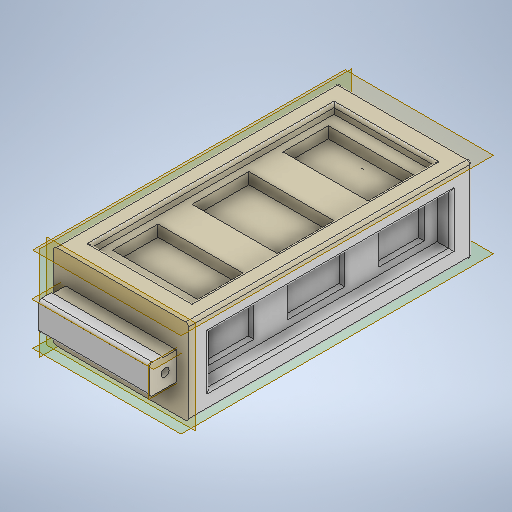
# Autodesk Inventor part: Part7
Saved by Autodesk Inventor 2025.2 (Build 292293000, 293)
## iProperties
Created: 2024-12-22
Part Number: Part7
Material: 一般
Document SubType Name: Modeling
Designer: mahhy
Density: 1 g/cm^3
Appearance: 既定
Author: mahhy
## iProperties of the stored document Part7_3D プリント.ipt
Created: 2024-12-23
Part Number: Part7_3D プリント
Material: 一般
Document SubType Name: Modeling
Designer: mahhy
Density: 1 g/cm^3
Appearance: 既定
Author: mahhy
Autodesk Inventor part; units mm, degrees
ref_plane "YZ Plane" through (0, 0, 0) normal (1, 0, 0) x (0, 1, 0)
ref_plane "XZ Plane" through (0, 0, 0) normal (0, 1, 0) x (-1, 0, 0)
ref_plane "XY Plane" through (0, 0, 0) normal (0, 0, 1) x (1, 0, 0)
sketch "スケッチ1" plane through (0, 0, 0) normal (0, 1, 0) x (-1, 0, 0)
  line L0 (0, 0) -> (47.5, 0)
  line L1 (47.5, 0) -> (47.5, -100)
  line L2 (47.5, -100) -> (0, -100)
  line L3 (0, -100) -> (0, 0)
  dimension "d0" = 47.5
  dimension "d1" = 100
  constraints: 8 end point, 2 parallel, 1 horizontal, 1 perpendicular
  measures "d0" distance of L1.end L2.end
  measures "d1" distance of L0.end L1.end
extrude "押し出し1" add sketch "スケッチ1" along normal blind 30
ref_plane "作業平面1" through (-47.5, 0, 0) normal (0, 0, 1) x (1, 0, 0)
sketch "スケッチ2" plane through (-47.5, 0, 0) normal (0, 0, 1) x (1, 0, 0)
  line L0 (4.25, 19.88) -> (43.25, 19.88)
  line L1 (43.25, 19.88) -> (43.25, 10.12)
  line L2 (43.25, 10.12) -> (4.25, 10.12)
  line L3 (4.25, 10.12) -> (4.25, 19.88)
  line L4 (47.5, 0) -> (0, 0) projected
  line L5 (0, 0) -> (47.5, 0) projected
  line L6 (0, 0) -> (0, 30) projected
  line L7 (0, 0) -> (0, 30) projected
  point P0 (23.75, 10.12)
  point P1 (23.75, 0)
  point P2 (23.75, 0)
  point P3 (4.25, 15)
  point P4 (0, 15)
  point P5 (0, 15)
  dimension "d5" = 39
  dimension "d6" = 9.76
  dimension "d7" = 0
  dimension "d8" = 0
  constraints: 8 end point, 6 midpoint, 2 parallel, 1 horizontal, 1 perpendicular
  measures "d5" distance of L1.end L2.end
  measures "d6" distance of L0.end L1.end
  measures "d7" horizontal distance of point (23.75, 0) point (23.75, 10.12)
  measures "d8" vertical distance of point (0, 15) point (4.25, 15)
extrude "押し出し2" add sketch "スケッチ2" along normal blind 9.5
ref_plane "作業平面2" through (-4.25, 10.12, 0) normal (1, 0, 0) x (0, 0, -1)
sketch "スケッチ3" plane through (-4.25, 10.12, 0) normal (1, 0, 0) x (0, 0, -1)
  line L0 (-9.5, 0) -> (-9.5, 9.76) projected
  line L1 (0, -10.12) -> (0, 19.88) projected
  point P0 (-9.5, 4.88)
  point P1 (-4, 4.88)
  point P2 (0, 4.88)
  dimension "d12" = 4
  constraints: 2 midpoint
  measures "d12" distance of point (0, 4.88) point (-4, 4.88)
hole "穴1" at (-4.25, 15, 4) direction (-1, 0, 0) diameter 2.85 end through all
ref_plane "作業平面3" through (-43.25, 19.88, 0) normal (0, 1, 0) x (1, 0, 0)
sketch "スケッチ4" plane through (-43.25, 19.88, 0) normal (0, 1, 0) x (1, 0, 0)
  line L0 (0, 0) -> (0, -9.5) projected
  line L1 (0, -9.5) -> (39, -9.5)
  line L2 (39, -9.5) -> (39, -5)
  line L3 (39, -5) -> (0, -5)
  line L4 (0, -5) -> (0, -9.5)
  point P0 (43.25, 0)
  dimension "d21" = 4.5
  constraints: 8 end point, 2 parallel, 1 horizontal, 1 perpendicular
  measures "d21" distance of L2.end L1.end
extrude "押し出し3" add sketch "スケッチ4" along normal blind 0.5
ref_plane "作業平面4" through (0, 30, 0) normal (0, 1, 0) x (1, 0, 0)
sketch "スケッチ6" plane through (0, 30, 0) normal (0, 1, 0) x (1, 0, 0)
  line L0 (-38.75, 28) -> (-8.75, 28)
  line L1 (-8.75, 28) -> (-8.75, 12)
  line L2 (-8.75, 12) -> (-38.75, 12)
  line L3 (-38.75, 12) -> (-38.75, 28)
  line L4 (-4.25, 0) -> (-43.25, 0) projected
  line L5 (9.5, 0) -> (-57, 0) projected
  line L6 (-38.75, 60) -> (-8.75, 60)
  line L7 (-8.75, 60) -> (-8.75, 40)
  line L8 (-8.75, 40) -> (-38.75, 40)
  line L9 (-38.75, 40) -> (-38.75, 60)
  line L10 (-38.75, 88) -> (-8.75, 88)
  line L11 (-8.75, 88) -> (-8.75, 72)
  line L12 (-8.75, 72) -> (-38.75, 72)
  line L13 (-38.75, 72) -> (-38.75, 88)
  line L14 (0, 100) -> (-47.5, 100) projected
  point P0 (0, 0)
  point P1 (-23.75, 12)
  point P2 (-23.75, 0)
  point P3 (-23.75, 40)
  point P4 (-23.75, 72)
  point P5 (-23.75, 60)
  point P6 (-23.75, 28)
  dimension "d37" = 30
  dimension "d38" = 16
  dimension "d39" = 0
  dimension "d40" = 12
  dimension "d41" = 30
  dimension "d42" = 20
  dimension "d43" = 30
  dimension "d44" = 16
  dimension "d45" = 12
  dimension "d46" = 12
  dimension "d47" = 12
  dimension "d48" = 0
  dimension "d49" = 0
  constraints: 24 end point, 6 midpoint, 6 parallel, 3 horizontal, 3 perpendicular
  measures "d37" distance of L1.end L2.end
  measures "d38" distance of L0.end L1.end
  measures "d39" horizontal distance of point (-23.75, 0) point (-23.75, 12)
  measures "d40" distance between parallel lines of L5 L2
  measures "d41" distance of L7.end L8.end
  measures "d42" distance of L6.end L7.end
  measures "d43" distance of L11.end L12.end
  measures "d44" distance of L10.end L11.end
  measures "d45" distance between parallel lines of L0 L8
  measures "d46" distance between parallel lines of L12 L6
  measures "d47" distance between parallel lines of L14 L10
  measures "d48" horizontal distance of point (-23.75, 60) point (-23.75, 72)
  measures "d49" horizontal distance of point (-23.75, 28) point (-23.75, 40)
extrude "押し出し5" cut sketch "スケッチ6" against normal blind 7
ref_plane "作業平面5" through (0, 0, 0) normal (0, -1, 0) x (1, 0, 0)
sketch "スケッチ7" plane through (0, 0, 0) normal (0, -1, 0) x (1, 0, 0)
  line L0 (-38.75, -72) -> (-8.75, -72)
  line L1 (-8.75, -72) -> (-8.75, -88)
  line L2 (-8.75, -88) -> (-38.75, -88)
  line L3 (-38.75, -88) -> (-38.75, -72)
  line L4 (-38.75, -40) -> (-8.75, -40)
  line L5 (-8.75, -40) -> (-8.75, -60)
  line L6 (-8.75, -60) -> (-38.75, -60)
  line L7 (-38.75, -60) -> (-38.75, -40)
  line L8 (-38.75, -12) -> (-8.75, -12)
  line L9 (-8.75, -12) -> (-8.75, -28)
  line L10 (-8.75, -28) -> (-38.75, -28)
  line L11 (-38.75, -28) -> (-38.75, -12)
  line L12 (-47.5, 0) -> (0, 0) projected
  point P0 (-23.75, -88)
  point P1 (-23.75, -60)
  point P2 (-23.75, -28)
  point P3 (-23.75, -40)
  point P4 (-23.75, -72)
  point P5 (-23.75, 0)
  point P6 (-23.75, -12)
  dimension "d53" = 30
  dimension "d54" = 16
  dimension "d55" = 30
  dimension "d56" = 20
  dimension "d57" = 30
  dimension "d58" = 16
  dimension "d59" = 12
  dimension "d60" = 12
  dimension "d61" = 0
  dimension "d62" = 0
  dimension "d63" = 0
  dimension "d64" = 12
  constraints: 24 end point, 7 midpoint, 6 parallel, 3 horizontal, 3 perpendicular
  measures "d53" distance of L1.end L3.start
  measures "d54" distance of L0.end L1.end
  measures "d55" distance of L6.start L6.end
  measures "d56" distance of L5.start L6.start
  measures "d57" distance of L10.start L10.end
  measures "d58" distance of L9.start L10.start
  measures "d59" distance between parallel lines of L0 L6
  measures "d60" distance between parallel lines of L10 L4
  measures "d61" horizontal distance of point (-23.75, -40) point (-23.75, -28)
  measures "d62" horizontal distance of point (-23.75, -72) point (-23.75, -60)
  measures "d63" horizontal distance of point (-23.75, 0) point (-23.75, -12)
  measures "d64" distance between parallel lines of L12 L8
extrude "押し出し6" cut sketch "スケッチ7" against normal blind 7
sketch "スケッチ8" plane through (0, 30, 0) normal (0, 1, 0) x (1, 0, 0)
  line L0 (-41.25, 92.5) -> (-6.25, 92.5)
  line L1 (-6.25, 92.5) -> (-6.25, 7.5)
  line L2 (-6.25, 7.5) -> (-41.25, 7.5)
  line L3 (-41.25, 7.5) -> (-41.25, 92.5)
  line L4 (0, 100) -> (-47.5, 100) projected
  line L5 (-47.5, 100) -> (-47.5, 0) projected
  line L6 (0, 0) -> (0, 100) projected
  point P0 (-23.75, 92.5)
  point P1 (-23.75, 100)
  point P2 (-41.25, 50)
  point P3 (-47.5, 50)
  dimension "d67" = 35
  dimension "d68" = 85
  dimension "d69" = 0
  dimension "d70" = 0
  dimension "d120" = 7.5
  dimension "d121" = 6.25
  constraints: 8 end point, 4 midpoint, 2 parallel, 1 horizontal, 1 perpendicular
  measures "d67" distance of L1.end L2.end
  measures "d68" distance of L0.end L1.end
  measures "d69" horizontal distance of point (-23.75, 100) point (-23.75, 92.5)
  measures "d70" vertical distance of point (-47.5, 50) point (-41.25, 50)
  measures "d120" distance between parallel lines of L4 L0
  measures "d121" distance between parallel lines of L6 L1
extrude "押し出し7" cut sketch "スケッチ8" against normal blind 3
sketch "スケッチ9" plane through (0, 0, 0) normal (0, -1, 0) x (1, 0, 0)
  line L0 (-6.25, -7.5) -> (-41.25, -7.5) projected
  line L1 (-6.25, -92.5) -> (-6.25, -7.5) projected
  line L2 (-41.25, -7.5) -> (-6.25, -7.5)
  line L3 (-6.25, -7.5) -> (-6.25, -92.5)
  line L4 (-6.25, -92.5) -> (-41.25, -92.5)
  line L5 (-41.25, -92.5) -> (-41.25, -7.5)
  point P0 (0, 0)
  constraints: 8 end point, 2 parallel, 1 horizontal, 1 perpendicular
extrude "押し出し8" cut sketch "スケッチ9" against normal blind 5
sketch "スケッチ10" plane through (0, 0, 0) normal (1, 0, 0) x (0, 0, -1)
  line L0 (0, 0) -> (100, 0) projected
  line L1 (0, 30) -> (100, 30) projected
  line L2 (100, 0) -> (100, 30) projected
  line L3 (0, 0) -> (0, 30) projected
  line L4 (88, 21.25) -> (72, 21.25)
  line L5 (72, 21.25) -> (72, 8.75)
  line L6 (72, 8.75) -> (88, 8.75)
  line L7 (88, 8.75) -> (88, 21.25)
  line L8 (60, 21.25) -> (40, 21.25)
  line L9 (40, 21.25) -> (40, 8.75)
  line L10 (40, 8.75) -> (60, 8.75)
  line L11 (60, 8.75) -> (60, 21.25)
  line L12 (28, 21.25) -> (12, 21.25)
  line L13 (12, 21.25) -> (12, 8.75)
  line L14 (12, 8.75) -> (28, 8.75)
  line L15 (28, 8.75) -> (28, 21.25)
  point P0 (100, 15)
  point P1 (12, 15)
  point P2 (80, 21.25)
  point P3 (50, 30)
  dimension "d82" = 16
  dimension "d83" = 20
  dimension "d84" = 16
  dimension "d85" = 12
  dimension "d86" = 12
  dimension "d87" = 12
  dimension "d88" = 12
  dimension "d90" = 8.75
  dimension "d91" = 8.75
  dimension "d92" = 8.75
  dimension "d93" = 8.75
  dimension "d94" = 8.75
  dimension "d95" = 8.75
  constraints: 24 end point, 6 parallel, 4 midpoint, 3 horizontal, 3 perpendicular
  measures "d82" distance of L6.end L5.end
  measures "d83" distance of L9.end L10.end
  measures "d84" distance of L13.end L14.end
  measures "d85" distance between parallel lines of L2 L7
  measures "d86" distance between parallel lines of L15 L9
  measures "d87" distance between parallel lines of L5 L11
  measures "d88" distance from line of L3 point (12, 15)
  measures "d90" distance from line of L1 point (80, 21.25)
  measures "d91" distance between parallel lines of L0 L6
  measures "d92" distance from line of point (50, 30) L8
  measures "d93" distance between parallel lines of L0 L10
  measures "d94" distance between parallel lines of L1 L12
  measures "d95" distance between parallel lines of L0 L14
extrude "押し出し9" cut sketch "スケッチ10" against normal blind 7 contours L7 L6 L5 L4 | L11 L10 L9 L8 | L15 L14 L13 L12
ref_plane "作業平面6" through (-47.5, 0, -100) normal (-1, 0, 0) x (0, 0, 1)
sketch "スケッチ12" plane through (-47.5, 0, -100) normal (-1, 0, 0) x (0, 0, 1)
  line L0 (88, 21.43) -> (72, 21.43)
  line L1 (72, 21.43) -> (72, 8.57)
  line L2 (72, 8.57) -> (88, 8.57)
  line L3 (88, 8.57) -> (88, 21.43)
  line L4 (60, 21.43) -> (40, 21.43)
  line L5 (40, 21.43) -> (40, 8.57)
  line L6 (40, 8.57) -> (60, 8.57)
  line L7 (60, 8.57) -> (60, 21.43)
  line L8 (28, 21.43) -> (12, 21.43)
  line L9 (12, 21.43) -> (12, 8.57)
  line L10 (12, 8.57) -> (28, 8.57)
  line L11 (28, 8.57) -> (28, 21.43)
  line L12 (0, 0) -> (0, 30) projected
  line L13 (-21.9, 30) -> (131.4, 30) projected
  line L14 (131.4, 0) -> (-21.9, 0) projected
  point P0 (100, 0)
  point P1 (12, 15)
  point P2 (80, 21.43)
  point P3 (0, 15)
  point P4 (0, 15)
  point P5 (40, 15)
  point P6 (72, 15)
  dimension "d101" = 16
  dimension "d102" = 20
  dimension "d103" = 16
  dimension "d104" = 12
  dimension "d105" = 12
  dimension "d106" = 0
  dimension "d107" = 0
  dimension "d108" = 0
  dimension "d109" = 12
  dimension "d111" = 8.57
  dimension "d112" = 8.57
  dimension "d113" = 8.57
  dimension "d114" = 8.57
  constraints: 24 end point, 6 midpoint, 6 parallel, 3 horizontal, 3 perpendicular
  measures "d101" distance of L2.end L1.end
  measures "d102" distance of L6.start L6.end
  measures "d103" distance of L9.end L11.start
  measures "d104" distance between parallel lines of L11 L5
  measures "d105" distance between parallel lines of L1 L7
  measures "d106" vertical distance of point (0, 15) point (12, 15)
  measures "d107" vertical distance of point (0, 15) point (40, 15)
  measures "d108" vertical distance of point (40, 15) point (72, 15)
  measures "d109" distance between parallel lines of L12 L9
  measures "d111" distance between parallel lines of L13 L8
  measures "d112" distance between parallel lines of L14 L10
  measures "d113" distance between parallel lines of L13 L4
  measures "d114" distance between parallel lines of L13 L0
extrude "押し出し11" cut sketch "スケッチ12" against normal blind 7
sketch "スケッチ14" plane through (-47.5, 0, -100) normal (-1, 0, 0) x (0, 0, 1)
  line L0 (7.5, 6.25) -> (92.5, 6.25)
  line L1 (92.5, 6.25) -> (92.5, 23.75)
  line L2 (92.5, 23.75) -> (7.5, 23.75)
  line L3 (7.5, 23.75) -> (7.5, 6.25)
  line L4 (0, 0) -> (0, 30) projected
  line L5 (100, 36) -> (100, -6) projected
  line L6 (-21.9, 30) -> (131.4, 30) projected
  line L7 (131.4, 0) -> (-21.9, 0) projected
  point P0 (100, 0)
  dimension "d127" = 7.5
  dimension "d128" = 7.5
  dimension "d129" = 6.25
  dimension "d130" = 6.25
  constraints: 8 end point, 2 parallel, 1 horizontal, 1 perpendicular
  measures "d127" distance between parallel lines of L4 L3
  measures "d128" distance between parallel lines of L5 L1
  measures "d129" distance between parallel lines of L6 L2
  measures "d130" distance between parallel lines of L7 L0
extrude "押し出し13" cut sketch "スケッチ14" against normal blind 5 contours L3 L2 L1 L0
sketch "スケッチ15" plane through (0, 0, 0) normal (1, 0, 0) x (0, 0, -1)
  line L0 (7.5, 23.75) -> (92.5, 23.75)
  line L1 (92.5, 23.75) -> (92.5, 6.25)
  line L2 (92.5, 6.25) -> (7.5, 6.25)
  line L3 (7.5, 6.25) -> (7.5, 23.75)
  line L4 (0, 0) -> (0, 30) projected
  line L5 (100, 0) -> (100, 30) projected
  line L6 (0, 30) -> (100, 30) projected
  line L7 (0, 0) -> (100, 0) projected
  dimension "d133" = 7.5
  dimension "d134" = 7.5
  dimension "d135" = 6.25
  dimension "d136" = 6.25
  constraints: 8 end point, 2 parallel, 1 horizontal, 1 perpendicular
  measures "d133" distance between parallel lines of L4 L3
  measures "d134" distance between parallel lines of L5 L1
  measures "d135" distance between parallel lines of L6 L0
  measures "d136" distance between parallel lines of L7 L2
extrude "押し出し14" cut sketch "スケッチ15" against normal blind 5 contours L0 L1 L2 L3
sketch "スケッチ16" plane through (0, 0, -100) normal (0, 0, -1) x (-1, 0, 0)
  line L0 (41.25, 0) -> (6.25, 0) projected
  line L1 (47.5, 0) -> (47.5, 30) projected
  circle A0 centre (23.75, 15) radius 1.75
  line L2 (0, 0) -> (47.5, 0) projected
  point P0 (23.75, 0)
  point P1 (47.5, 15)
  point P2 (23.75, 0)
  dimension "d139" = 3.5
  dimension "d153" = 0
  dimension "d154" = 0
  constraints: 3 midpoint, 1 centre point, 1 coincident
  measures "d139" diameter of A0
  measures "d153" vertical distance of A0.centre point (47.5, 15)
  measures "d154" horizontal distance of point (23.75, 0) A0.centre
extrude "押し出し15" cut sketch "スケッチ16" against normal blind 7
sketch "スケッチ17" plane through (0, 0, -100) normal (0, 0, -1) x (-1, 0, 0)
  line L0 (-9.5, 30) -> (57, 30) projected
  line L1 (0, 0) -> (47.5, 0) projected
  line L2 (0, 0) -> (0, 30) projected
  line L3 (47.5, 36) -> (47.5, -6) projected
  point P0 (23.75, 21.5)
  point P1 (23.75, 8.5)
  point P2 (14, 15.1266)
  point P3 (33.5, 15.1266)
  point P4 (0, 15)
  dimension "d142" = 8.5
  dimension "d143" = 8.5
  dimension "d144" = 14
  dimension "d145" = 14
  dimension "d155" = 19.5
  constraints: 1 midpoint
  measures "d142" distance from line of L0 point (23.75, 21.5)
  measures "d143" distance from line of L1 point (23.75, 8.5)
  measures "d144" horizontal distance of point (0, 15) point (14, 15.127)
  measures "d145" distance from line of L3 point (33.5, 15.127)
  measures "d155" distance of point (33.5, 15.127) point (14, 15.127)
hole "穴2" at (-23.75, 21.5, -100) at (-23.75, 8.5, -100) at (-14, 15.1266, -100) at (-33.5, 15.1266, -100) direction (0, 0, 1) diameter 2.85 depth 15 tip angle 118
fillet "フィレット1" radius 1 1 edges at (-23.75, 30, -100)
fillet "フィレット1" radius 1 23 edges at (0, 30, -50) (-47.5, 30, -50) (0, 15, -92.5) (0, 6.25, -50) (0, 23.75, -50) (0, 15, -7.5) (-41.25, 30, -50) (-23.75, 30, -92.5) (-23.75, 30, -7.5) (-6.25, 30, -50) (0, 0, -50) (0, 15, -100) (-47.5, 15, -100) (-47.5, 0, -50) (-6.25, 0, -50) (-23.75, 0, -92.5) (-41.25, 0, -50) (-23.75, 0, -7.5) (-23.75, 0, -100) (-47.5, 15, -7.5) (-47.5, 6.25, -50) (-47.5, 23.75, -50) (-47.5, 15, -92.5)
fillet "フィレット2" radius 1 2 edges at (-23.75, 10.12, 9.5) (-23.75, 20.38, 9.5)
